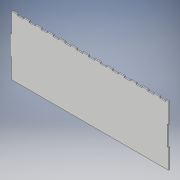
# Autodesk Inventor part: Pared1
Saved by Autodesk Inventor 2019 (Build 230136000, 136)
## iProperties
Created: 2020-03-08
Part Number: Pared1
Material: Genérico
Document SubType Name: Modeling
Designer: Diego Guillén
Density: 1 g/cm^3
Appearance: Valor por defecto
Author: Diego Guillén
Autodesk Inventor part; units mm, degrees
ref_plane "YZ Plane" through (0, 0, 0) normal (1, 0, 0) x (0, 1, 0)
ref_plane "XZ Plane" through (0, 0, 0) normal (0, 1, 0) x (-1, 0, 0)
ref_plane "XY Plane" through (0, 0, 0) normal (0, 0, 1) x (1, 0, 0)
sketch "Boceto1" plane through (0, 0, 0) normal (0, 0, 1) x (1, 0, 0)
  line L0 (0, 0) -> (400, 0)
  line L1 (400, 0) -> (400, 150)
  line L2 (400, 150) -> (0, 150)
  line L3 (0, 150) -> (0, 0)
  dimension "d0" = 150
  dimension "d1" = 400
  constraints: 8 end point, 2 parallel, 1 horizontal, 1 perpendicular
  measures "d0" distance of L0.end L1.end
  measures "d1" distance of L1.end L2.end
extrude "Extrusión1" add sketch "Boceto1" along normal blind 3
sketch "Boceto3" plane through (0, 0, 3) normal (0, 0, 1) x (1, 0, 0)
  line L0 (0, 0) -> (400, 0) construction
  line L1 (400, 0) -> (400, 150) construction
  line L2 (400, 150) -> (0, 150) construction
  line L3 (0, 150) -> (0, 0) construction
  line L4 (0, 50) -> (3, 50)
  line L5 (3, 50) -> (3, 0)
  line L6 (3, 0) -> (0, 0)
  line L7 (0, 0) -> (0, 50)
  line L8 (0, 100) -> (0, 150)
  line L9 (0, 150) -> (3, 150)
  line L10 (3, 150) -> (3, 100)
  line L11 (3, 100) -> (0, 100)
  line L12 (397, 100) -> (400, 100)
  line L13 (400, 100) -> (400, 50)
  line L14 (400, 50) -> (397, 50)
  line L15 (397, 50) -> (397, 100)
  line L16 (400, 0) -> (400, 150) construction
  point P0 (400, 75)
  point P1 (400, 75)
  dimension "d15" = 3
  dimension "d16" = 50
  dimension "d19" = 100
  dimension "d24" = 3
  dimension "d25" = 50
  constraints: 24 end point, 4 parallel, 2 coincident, 2 horizontal, 2 midpoint, 2 perpendicular, 1 collinear, 1 vertical, 8 other
  measures "d15" distance of L5.end L6.end
  measures "d16" distance of L4.end L5.end
  measures "d19" distance of L6.end L8.start
  measures "d24" distance of L13.end L14.end
  measures "d25" distance of L14.end L12.start
extrude "Extrusión3" cut sketch "Boceto3" against normal blind 3
sketch "Boceto4" plane through (0, 0, 3) normal (0, 0, 1) x (1, 0, 0)
  line L0 (3, 150) -> (3, 100) construction
  line L1 (3, 100) -> (0, 100) construction
  line L2 (0, 100) -> (0, 50) construction
  line L3 (0, 50) -> (3, 50) construction
  line L4 (3, 50) -> (3, 0) construction
  line L5 (3, 0) -> (400, 0) construction
  line L6 (400, 0) -> (400, 50) construction
  line L7 (400, 50) -> (397, 50) construction
  line L8 (397, 50) -> (397, 100) construction
  line L9 (397, 100) -> (400, 100) construction
  line L10 (400, 100) -> (400, 150) construction
  line L11 (400, 150) -> (3, 150) construction
  line L12 (18, 150) -> (33, 150)
  line L13 (33, 150) -> (33, 147)
  line L14 (33, 147) -> (18, 147)
  line L15 (18, 147) -> (18, 150)
  line L16 (3, 0) -> (400, 0) construction
  line L17 (63, 147) -> (48, 147)
  line L18 (48, 147) -> (48, 150)
  line L19 (48, 150) -> (63, 150)
  line L20 (63, 150) -> (63, 147)
  line L21 (93, 147) -> (78, 147)
  line L22 (78, 147) -> (78, 150)
  line L23 (78, 150) -> (93, 150)
  line L24 (93, 150) -> (93, 147)
  line L25 (123, 147) -> (108, 147)
  line L26 (108, 147) -> (108, 150)
  line L27 (108, 150) -> (123, 150)
  line L28 (123, 150) -> (123, 147)
  line L29 (153, 147) -> (138, 147)
  line L30 (138, 147) -> (138, 150)
  line L31 (138, 150) -> (153, 150)
  line L32 (153, 150) -> (153, 147)
  line L33 (183, 147) -> (168, 147)
  line L34 (168, 147) -> (168, 150)
  line L35 (168, 150) -> (183, 150)
  line L36 (183, 150) -> (183, 147)
  line L37 (213, 147) -> (198, 147)
  line L38 (198, 147) -> (198, 150)
  line L39 (198, 150) -> (213, 150)
  line L40 (213, 150) -> (213, 147)
  line L41 (243, 147) -> (228, 147)
  line L42 (228, 147) -> (228, 150)
  line L43 (228, 150) -> (243, 150)
  line L44 (243, 150) -> (243, 147)
  line L45 (273, 147) -> (258, 147)
  line L46 (258, 147) -> (258, 150)
  line L47 (258, 150) -> (273, 150)
  line L48 (273, 150) -> (273, 147)
  line L49 (303, 147) -> (288, 147)
  line L50 (288, 147) -> (288, 150)
  line L51 (288, 150) -> (303, 150)
  line L52 (303, 150) -> (303, 147)
  line L53 (333, 147) -> (318, 147)
  line L54 (318, 147) -> (318, 150)
  line L55 (318, 150) -> (333, 150)
  line L56 (333, 150) -> (333, 147)
  line L57 (363, 147) -> (348, 147)
  line L58 (348, 147) -> (348, 150)
  line L59 (348, 150) -> (363, 150)
  line L60 (363, 150) -> (363, 147)
  line L61 (393, 147) -> (378, 147)
  line L62 (378, 147) -> (378, 150)
  line L63 (378, 150) -> (393, 150)
  line L64 (393, 150) -> (393, 147)
  line L65 (400, 150) -> (3, 150) construction
  point P0 (0, 0)
  dimension "d28" = 3
  dimension "d29" = 15
  dimension "d30" = 15
  dimension "d33" = 30
  constraints: 104 end point, 2 horizontal, 2 parallel, 1 collinear, 1 perpendicular, 96 other
  measures "d28" distance of L14.end L12.start
  measures "d29" distance of L12.start L12.end
  measures "d30" distance from line of L4 L12.start
  measures "d33" distance of L13.end L17.start
extrude "Extrusión4" cut sketch "Boceto4" against normal blind 10
